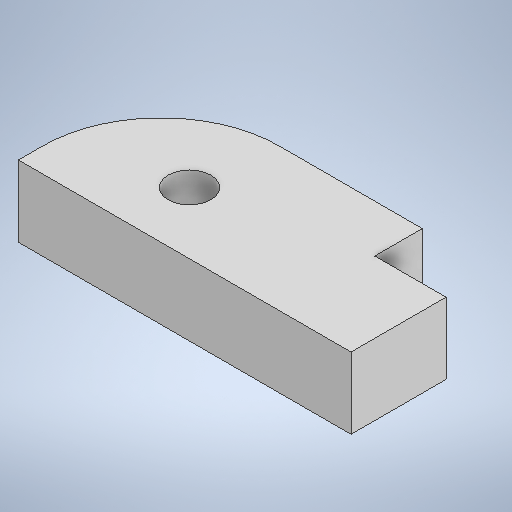
# Autodesk Inventor part: SoporteServo
Saved by Autodesk Inventor 2025.2 (Build 292293000, 293)
## iProperties
Created: 2025-03-05
Part Number: SoporteServo
Material: Generic
Document SubType Name: Modeling
Designer: cdavi
Density: 1 g/cm^3
Appearance: Default
Author: cdavi
Autodesk Inventor part; units mm, degrees
ref_plane "YZ Plane" through (0, 0, 0) normal (1, 0, 0) x (0, 1, 0)
ref_plane "XZ Plane" through (0, 0, 0) normal (0, 1, 0) x (-1, 0, 0)
ref_plane "XY Plane" through (0, 0, 0) normal (0, 0, 1) x (1, 0, 0)
sketch "Sketch1" plane through (0, 0, 0) normal (0, 1, 0) x (-1, 0, 0)
  line L0 (0, 0) -> (0, -4)
  line L1 (0, -4) -> (3, -4)
  line L2 (3, -4) -> (3, -6)
  line L3 (3, -6) -> (9, -6)
  line L4 (14, -1) -> (14, 0)
  line L5 (14, 0) -> (0, 0)
  circle A0 centre (9.4, -2.6) radius 0.9
  arc A1 (9, -6) -> (14, -1) centre (9, -1) ccw
  dimension "d1" = 6
  dimension "d2" = 2
  dimension "d3" = 3
  dimension "d4" = 14
  dimension "d5" = 2.6
  dimension "d6" = 4.6
  dimension "d7" = 1.8
  dimension "d8" = 5
  constraints: 12 end point, 5 perpendicular, 2 centre point, 2 point on circle, 2 tangent, 1 vertical
  measures "d1" distance between parallel lines of L3 L5
  measures "d2" distance of L1.end L2.end
  measures "d3" distance of L0.end L1.end
  measures "d4" distance between parallel lines of L0 L4
  measures "d5" vertical distance of L0.start A0.centre
  measures "d6" distance from line of A0.centre L4
  measures "d7" diameter of A0
  measures "d8" radius of A1
extrude "Extrusion1" add sketch "Sketch1" along normal blind 3
body "Solid1"
